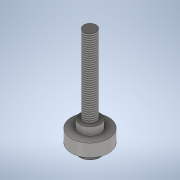
# Autodesk Inventor part: rod and bearing
Saved by Autodesk Inventor 2021 (Build 250183000, 183)
## iProperties
Created: 2021-07-30
Part Number: rod and bearing
Material: Stainless Steel
Document SubType Name: Modeling
Designer: samlo
Density: 8 g/cm^3
Appearance: Steel - Polished
Author: samlo
Autodesk Inventor part; units mm, degrees
ref_plane "YZ Plane" through (0, 0, 0) normal (1, 0, 0) x (0, 1, 0)
ref_plane "XZ Plane" through (0, 0, 0) normal (0, 1, 0) x (-1, 0, 0)
ref_plane "XY Plane" through (0, 0, 0) normal (0, 0, 1) x (1, 0, 0)
sketch "Sketch1" plane through (0, 0, 0) normal (0, 0, 1) x (1, 0, 0)
  line L0 (0, 0) -> (6.5, 0)
  line L1 (6.5, 0) -> (6.5, 5.13)
  line L2 (6.5, 5.13) -> (11.99, 5.13)
  line L3 (11.99, 5.13) -> (11.99, 13.25)
  line L4 (11.99, 13.25) -> (6.5, 13.25)
  line L5 (6.5, 13.25) -> (6.5, 18.38)
  line L6 (6.5, 18.38) -> (4, 18.38)
  line L7 (4, 18.38) -> (4, 68.95)
  line L8 (4, 68.95) -> (0, 68.95)
  line L9 (0, 68.95) -> (0, 0)
  dimension "d0" = 4
  dimension "d2" = 68.95
  dimension "d3" = 8.12
  dimension "d4" = 5.13
  dimension "d5" = 5.13
  dimension "d6" = 11.99
  dimension "d7" = 6.5
  constraints: 20 end point, 8 perpendicular, 2 point on line, 1 horizontal
  measures "d0" distance of L7.end L8.end
  measures "d2" distance of L8.end L0.start
  measures "d3" distance of L2.end L3.end
  measures "d4" distance of L0.end L1.end
  measures "d5" distance of L4.end L5.end
  measures "d6" distance from line of L3 L0.start
  measures "d7" distance of L0.start L0.end
revolve "Revolution1" add sketch "Sketch1" angle 360 about axis through (0, 68.95, 0) along (0, -1, 0)
thread "Thread1" size "M8x1.25" class "6g" standard "ANSI Metric M Profile" full length
body "Solid1"
